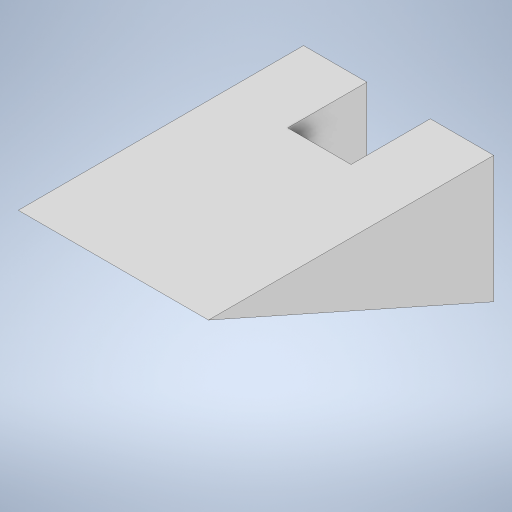
# Autodesk Inventor part: Tapered
Saved by Autodesk Inventor 2024 (Build 280153000, 153)
## iProperties
Created: 2023-12-21
Part Number: Tapered
Material: Generic
Document SubType Name: Modeling
Designer: pratikhya
Density: 1 g/cm^3
Appearance: Default
Author: pratikhya
Autodesk Inventor part; units mm, degrees
ref_plane "YZ Plane" through (0, 0, 0) normal (1, 0, 0) x (0, 1, 0)
ref_plane "XZ Plane" through (0, 0, 0) normal (0, 1, 0) x (-1, 0, 0)
ref_plane "XY Plane" through (0, 0, 0) normal (0, 0, 1) x (1, 0, 0)
sketch "Sketch1" plane through (0, 0, 0) normal (0, 0, 1) x (1, 0, 0)
  point P0 (0, 0)
sketch "Sketch2" plane through (0, 0, 0) normal (1, 0, 0) x (0, 1, 0)
  line L0 (3.3322, 3.9709) -> (123.3322, 3.9709) construction
  line L1 (3.3322, 3.9709) -> (3.3322, -266.0291)
  line L2 (-116.6678, -266.0291) -> (3.3322, -266.0291)
  line L3 (3.3322, 3.9709) -> (-116.6678, -266.0291)
  point P0 (0, 0)
  dimension "d6" = 270
  constraints: 8 end point, 1 horizontal, 1 vertical
  measures "d6" distance of L0.start L1.end
extrude "Extrusion1" add sketch "Sketch2" along normal blind 180
sketch "Sketch3" plane through (0, 3.3322, 3.9709) normal (0, 1, 0) x (1, 0, 0)
  line L0 (0, 0) -> (0, 270) projected
  line L1 (0, 270) -> (60, 270)
  line L2 (0, 270) -> (180, 270) projected
  line L3 (60, 270) -> (120, 270)
  line L4 (120, 270) -> (180, 270)
  line L5 (60, 270) -> (60, 195)
  line L6 (60, 195) -> (120, 195)
  line L7 (120, 195) -> (120, 270)
  point P0 (0, 3.9709)
  dimension "d7" = 60
  dimension "d8" = 60
  dimension "d9" = 75
  constraints: 12 end point, 2 perpendicular, 2 point on line, 1 collinear, 1 vertical
  measures "d7" distance of L0.end L1.end
  measures "d8" distance of L1.end L3.end
  measures "d9" distance of L1.end L5.end
extrude "Extrusion2" cut sketch "Sketch3" against normal blind 191.475
body "Solid1"
